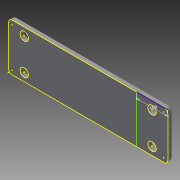
# Autodesk Inventor part: spacer plate
Saved by Autodesk Inventor 2013 (Build 170138000, 138)
## iProperties
Created: 2013-02-04
Part Number: spacer plate
Material: Generic
Document SubType Name: Modeling
Designer: Arpan
Density: 1 g/cm^3
Author: Arpan
Autodesk Inventor part; units mm, degrees
ref_plane "YZ Plane" through (0, 0, 0) normal (1, 0, 0) x (0, 1, 0)
ref_plane "XZ Plane" through (0, 0, 0) normal (0, 1, 0) x (-1, 0, 0)
ref_plane "XY Plane" through (0, 0, 0) normal (0, 0, 1) x (1, 0, 0)
sketch "Sketch1" plane through (0, 0, 0) normal (0, 0, 1) x (1, 0, 0)
  line L0 (0, 0) -> (0, 38.1)
  line L1 (0, 38.1) -> (128.1684, 38.1)
  line L2 (128.1684, 38.1) -> (128.1684, 0)
  line L3 (128.1684, 0) -> (0, 0)
  dimension "d0" = 38.1
  dimension "d1" = 128.1684
  constraints: 8 end point, 2 perpendicular, 1 parallel, 1 vertical
  measures "d0" distance of L0.start L0.end
  measures "d1" distance of L0.end L1.end
extrude "Extrusion1" add sketch "Sketch1" along normal blind 3.175
sketch "Sketch2" plane through (0, 0, 3.175) normal (0, 0, 1) x (1, 0, 0)
  line L0 (128.1684, 38.1) -> (0, 38.1) projected
  line L1 (0, 38.1) -> (12.7, 38.1)
  line L2 (12.7, 38.1) -> (12.7, 31.75)
  line L3 (12.7, 31.75) -> (12.7, 6.35)
  circle A0 centre (12.7, 31.75) radius 3.3782
  circle A1 centre (12.7, 6.35) radius 3.3782
  line L4 (128.1684, 38.1) -> (115.4684, 38.1)
  line L5 (115.4684, 38.1) -> (115.4684, 31.75)
  circle A2 centre (115.4684, 31.75) radius 3.3782
  circle A3 centre (115.4684, 6.35) radius 3.3782
  line L6 (115.4684, 6.35) -> (115.4684, 31.75)
  dimension "d4" = 12.7
  dimension "d5" = 6.35
  dimension "d6" = 25.4
  dimension "d7" = 6.7564
  dimension "d8" = 6.7564
  dimension "d9" = 12.7
  dimension "d10" = 6.35
  dimension "d11" = 6.7564
  dimension "d12" = 6.7564
  dimension "d13" = 25.4
  constraints: 12 end point, 4 centre point, 3 coincident, 2 collinear, 2 perpendicular, 2 point on line
  measures "d4" distance of L0.end L1.end
  measures "d5" distance of L1.end L2.end
  measures "d6" distance of L2.end L3.end
  measures "d7" diameter of A0
  measures "d8" diameter of A1
  measures "d9" distance of L0.start L4.end
  measures "d10" distance of L4.end L5.end
  measures "d11" diameter of A2
  measures "d12" diameter of A3
  measures "d13" distance of L6.start L6.end
extrude "Extrusion2" cut sketch "Sketch2" against normal blind 3.175
fillet "Fillet1" radius 3.175 4 edges at (128.1684, 38.1, 1.5875) (128.1684, 0, 1.5875) (0, 38.1, 1.5875) (0, 0, 1.5875)
sketch "Sketch3" plane through (0, 0, 3.175) normal (0, 0, 1) x (1, 0, 0)
  arc A0 (0, 3.175) -> (3.175, 0) centre (3.175, 3.175) ccw projected
  line L0 (3.175, 0) -> (124.9934, 0) projected
  arc A1 (124.9934, 0) -> (128.1684, 3.175) centre (124.9934, 3.175) ccw projected
  line L1 (128.1684, 3.175) -> (128.1684, 34.925) projected
  arc A2 (128.1684, 34.925) -> (124.9934, 38.1) centre (124.9934, 34.925) ccw projected
  line L2 (124.9934, 38.1) -> (3.175, 38.1) projected
  arc A3 (3.175, 38.1) -> (0, 34.925) centre (3.175, 34.925) ccw projected
  line L3 (0, 34.925) -> (0, 3.175) projected
  circle A4 centre (115.4684, 31.75) radius 3.3782 projected
  circle A5 centre (12.7, 31.75) radius 3.3782 projected
  circle A6 centre (12.7, 6.35) radius 3.3782 projected
  circle A7 centre (115.4684, 6.35) radius 3.3782 projected
  line L4 (128.1684, 38.1) -> (102.7684, 38.1)
  line L5 (102.7684, 38.1) -> (102.7684, 0)
  point P0 (0, 0)
  dimension "d17" = 25.4
  constraints: 4 end point, 3 point on line, 1 perpendicular
  measures "d17" distance of L4.start L4.end
body "Solid1"
